Autodesk Inventor part; units mm, degrees
(part 2 of 4)
  line L790 (-24.261051, 21.500592) -> (-24.576272, 21.93055)
  line L791 (-24.576272, 21.93055) -> (-24.635193, 21.981033)
  line L792 (-24.635193, 21.981033) -> (-24.227981, 22.446234)
  line L793 (-24.227981, 22.446234) -> (-22.535064, 20.962239)
  line L794 (-22.535064, 20.962239) -> (-22.945382, 20.499895)
  line L795 (-22.945382, 20.499895) -> (-23.011524, 20.555712)
  line L796 (-23.011524, 20.555712) -> (-23.5045, 20.83708)
  line L797 (-23.5045, 20.83708) -> (-23.53757, 20.838033)
  line L798 (-23.53757, 20.838033) -> (-23.570641, 20.839176)
  line L799 (-23.570641, 20.839176) -> (-23.969586, 20.579524)
  line L800 (-23.969586, 20.579524) -> (-24.016106, 20.525803)
  line L801 (-24.016106, 20.525803) -> (-24.095678, 20.433792)
  line L802 (-24.095678, 20.433792) -> (-22.899891, 19.386042)
  line L803 (-22.899891, 19.386042) -> (-22.46477, 19.882866)
  line L804 (-22.46477, 19.882866) -> (-22.375901, 19.985355)
  line L805 (-22.375901, 19.985355) -> (-22.068949, 20.441221)
  line L806 (-22.068949, 20.441221) -> (-21.949048, 20.82565)
  line L807 (-21.949048, 20.82565) -> (-21.952134, 20.891754)
  line L808 (-21.952134, 20.891754) -> (-21.956287, 20.959)
  line L809 (-21.956287, 20.959) -> (-22.111316, 21.344382)
  line L810 (-22.111316, 21.344382) -> (-22.449282, 21.799296)
  line L811 (-22.449282, 21.799296) -> (-22.543313, 21.900261)
  line L812 (-22.543313, 21.900261) -> (-22.117507, 22.386036)
  line L813 (-22.117507, 22.386036) -> (-20.586859, 21.043582)
  line L814 (-20.586859, 21.043582) -> (-23.801127, 17.377791)
  line L815 (-19.514058, 26.962608) -> (-19.53888, 27.003184)
  line L816 (-19.53888, 27.003184) -> (-19.754869, 27.21483)
  line L817 (-19.754869, 27.21483) -> (-19.772452, 27.217878)
  line L818 (-19.772452, 27.217878) -> (-19.791045, 27.221116)
  line L819 (-19.791045, 27.221116) -> (-20.087673, 27.107388)
  line L820 (-20.087673, 27.107388) -> (-20.127963, 27.08148)
  line L821 (-20.127963, 27.08148) -> (-20.346029, 26.942986)
  line L822 (-20.346029, 26.942986) -> (-20.691234, 27.489722)
  line L823 (-20.691234, 27.489722) -> (-18.695479, 28.747593)
  line L824 (-18.695479, 28.747593) -> (-15.261145, 26.846974)
  line L825 (-15.261145, 26.846974) -> (-16.523017, 28.848939)
  line L826 (-16.523017, 28.848939) -> (-16.547782, 28.889325)
  line L827 (-16.547782, 28.889325) -> (-16.763809, 29.10097)
  line L828 (-16.763809, 29.10097) -> (-16.781336, 29.104209)
  line L829 (-16.781336, 29.104209) -> (-16.800004, 29.107257)
  line L830 (-16.800004, 29.107257) -> (-17.096613, 28.993528)
  line L831 (-17.096613, 28.993528) -> (-17.136999, 28.967621)
  line L832 (-17.136999, 28.967621) -> (-17.3736, 28.817887)
  line L833 (-17.3736, 28.817887) -> (-17.717833, 29.364432)
  line L834 (-17.717833, 29.364432) -> (-15.813024, 30.565534)
  line L835 (-15.813024, 30.565534) -> (-15.46879, 30.018799)
  line L836 (-15.46879, 30.018799) -> (-15.663101, 29.895736)
  line L837 (-15.663101, 29.895736) -> (-15.704439, 29.870209)
  line L838 (-15.704439, 29.870209) -> (-15.934944, 29.652849)
  line L839 (-15.934944, 29.652849) -> (-15.940087, 29.63437)
  line L840 (-15.940087, 29.63437) -> (-15.945231, 29.616844)
  line L841 (-15.945231, 29.616844) -> (-15.84598, 29.331475)
  line L842 (-15.84598, 29.331475) -> (-15.821215, 29.29128)
  line L843 (-15.821215, 29.29128) -> (-13.762482, 26.0263)
  line L844 (-13.762482, 26.0263) -> (-15.043976, 25.218962)
  line L845 (-15.043976, 25.218962) -> (-18.71091, 27.243786)
  line L846 (-18.71091, 27.243786) -> (-17.326165, 25.048654)
  line L847 (-17.326165, 25.048654) -> (-17.30121, 25.009221)
  line L848 (-17.30121, 25.009221) -> (-17.087278, 24.796432)
  line L849 (-17.087278, 24.796432) -> (-17.0688, 24.793385)
  line L850 (-17.0688, 24.793385) -> (-17.051083, 24.790146)
  line L851 (-17.051083, 24.790146) -> (-16.754475, 24.905018)
  line L852 (-16.754475, 24.905018) -> (-16.713136, 24.929783)
  line L853 (-16.713136, 24.929783) -> (-16.476535, 25.079515)
  line L854 (-16.476535, 25.079515) -> (-16.131349, 24.532971)
  line L855 (-16.131349, 24.532971) -> (-18.059781, 23.317391)
  line L856 (-18.059781, 23.317391) -> (-18.405157, 23.864126)
  line L857 (-18.405157, 23.864126) -> (-18.185892, 24.001666)
  line L858 (-18.185892, 24.001666) -> (-18.145696, 24.027575)
  line L859 (-18.145696, 24.027575) -> (-17.914239, 24.245697)
  line L860 (-17.914239, 24.245697) -> (-17.908905, 24.263032)
  line L861 (-17.908905, 24.263032) -> (-17.904904, 24.280749)
  line L862 (-17.904904, 24.280749) -> (-18.003012, 24.56707)
  line L863 (-18.003012, 24.56707) -> (-18.027777, 24.606313)
  line L864 (-18.027777, 24.606313) -> (-19.514058, 26.962608)
  line L865 (-10.748772, 31.507176) -> (-10.761154, 31.552705)
  line L866 (-10.761154, 31.552705) -> (-10.903649, 31.819405)
  line L867 (-10.903649, 31.819405) -> (-10.920222, 31.826454)
  line L868 (-10.920222, 31.826454) -> (-10.936796, 31.835788)
  line L869 (-10.936796, 31.835788) -> (-11.253025, 31.814071)
  line L870 (-11.253025, 31.814071) -> (-11.299507, 31.800546)
  line L871 (-11.299507, 31.800546) -> (-11.549634, 31.73368)
  line L872 (-11.549634, 31.73368) -> (-11.717083, 32.357758)
  line L873 (-11.717083, 32.357758) -> (-9.440418, 32.971549)
  line L874 (-9.440418, 32.971549) -> (-6.717982, 30.143958)
  line L875 (-6.717982, 30.143958) -> (-7.334059, 32.428053)
  line L876 (-7.334059, 32.428053) -> (-7.346442, 32.473392)
  line L877 (-7.346442, 32.473392) -> (-7.488936, 32.740092)
  line L878 (-7.488936, 32.740092) -> (-7.50551, 32.748283)
  line L879 (-7.50551, 32.748283) -> (-7.522083, 32.756665)
  line L880 (-7.522083, 32.756665) -> (-7.838313, 32.734948)
  line L881 (-7.838313, 32.734948) -> (-7.884795, 32.721613)
  line L882 (-7.884795, 32.721613) -> (-8.155495, 32.649033)
  line L883 (-8.155495, 32.649033) -> (-8.324088, 33.273492)
  line L884 (-8.324088, 33.273492) -> (-6.150483, 33.85947)
  line L885 (-6.150483, 33.85947) -> (-5.98189, 33.235201)
  line L886 (-5.98189, 33.235201) -> (-6.203061, 33.175384)
  line L887 (-6.203061, 33.175384) -> (-6.250686, 33.162811)
  line L888 (-6.250686, 33.162811) -> (-6.536055, 33.023365)
  line L889 (-6.536055, 33.023365) -> (-6.545199, 33.007744)
  line L890 (-6.545199, 33.007744) -> (-6.555486, 32.992314)
  line L891 (-6.555486, 32.992314) -> (-6.545199, 32.689609)
  line L892 (-6.545199, 32.689609) -> (-6.532816, 32.64408)
  line L893 (-6.532816, 32.64408) -> (-5.527358, 28.91809)
  line L894 (-5.527358, 28.91809) -> (-6.990779, 28.523375)
  line L895 (-6.990779, 28.523375) -> (-9.897046, 31.540132)
  line L896 (-9.897046, 31.540132) -> (-9.221343, 29.032771)
  line L897 (-9.221343, 29.032771) -> (-9.209913, 28.988575)
  line L898 (-9.209913, 28.988575) -> (-9.066276, 28.721876)
  line L899 (-9.066276, 28.721876) -> (-9.049512, 28.713303)
  line L900 (-9.049512, 28.713303) -> (-9.034272, 28.705111)
  line L901 (-9.034272, 28.705111) -> (-8.717661, 28.726828)
  line L902 (-8.717661, 28.726828) -> (-8.670417, 28.739401)
  line L903 (-8.670417, 28.739401) -> (-8.399526, 28.812553)
  line L904 (-8.399526, 28.812553) -> (-8.230933, 28.188475)
  line L905 (-8.230933, 28.188475) -> (-10.432542, 27.595258)
  line L906 (-10.432542, 27.595258) -> (-10.600753, 28.218384)
  line L907 (-10.600753, 28.218384) -> (-10.35177, 28.286583)
  line L908 (-10.35177, 28.286583) -> (-10.305288, 28.300108)
  line L909 (-10.305288, 28.300108) -> (-10.020109, 28.439554)
  line L910 (-10.020109, 28.439554) -> (-10.009632, 28.454033)
  line L911 (-10.009632, 28.454033) -> (-10.000488, 28.469653)
  line L912 (-10.000488, 28.469653) -> (-10.010775, 28.772358)
  line L913 (-10.010775, 28.772358) -> (-10.022205, 28.816744)
  line L914 (-10.022205, 28.816744) -> (-10.748772, 31.507176)
  line L915 (-1.875853, 29.406151) -> (-1.860232, 30.051946)
  line L916 (-1.860232, 30.051946) -> (-1.587436, 30.04585)
  line L917 (-1.587436, 30.04585) -> (-1.539811, 30.044707)
  line L918 (-1.539811, 30.044707) -> (-1.231963, 30.096333)
  line L919 (-1.231963, 30.096333) -> (-1.217676, 30.107763)
  line L920 (-1.217676, 30.107763) -> (-1.20415, 30.120145)
  line L921 (-1.20415, 30.120145) -> (-1.129855, 30.414658)
  line L922 (-1.129855, 30.414658) -> (-1.128712, 30.46114)
  line L923 (-1.128712, 30.46114) -> (-1.060513, 33.246441)
  line L924 (-1.060513, 33.246441) -> (-1.05937, 33.295209)
  line L925 (-1.05937, 33.295209) -> (-1.119188, 33.594865)
  line L926 (-1.119188, 33.594865) -> (-1.13157, 33.606295)
  line L927 (-1.13157, 33.606295) -> (-1.145095, 33.618678)
  line L928 (-1.145095, 33.618678) -> (-1.451038, 33.683829)
  line L929 (-1.451038, 33.683829) -> (-1.498663, 33.684972)
  line L930 (-1.498663, 33.684972) -> (-1.770316, 33.69202)
  line L931 (-1.770316, 33.69202) -> (-1.754886, 34.337815)
  line L932 (-1.754886, 34.337815) -> (3.119247, 34.217991)
  line L933 (3.119247, 34.217991) -> (3.073718, 32.337184)
  line L934 (3.073718, 32.337184) -> (2.42678, 32.353568)
  line L935 (2.42678, 32.353568) -> (2.418588, 32.425957)
  line L936 (2.418588, 32.425957) -> (2.311908, 32.971549)
  line L937 (2.311908, 32.971549) -> (2.299526, 33.007744)
  line L938 (2.299526, 33.007744) -> (2.286191, 33.045082)
  line L939 (2.286191, 33.045082) -> (2.11055, 33.339595)
  line L940 (2.11055, 33.339595) -> (2.088832, 33.360169)
  line L941 (2.088832, 33.360169) -> (2.066163, 33.383029)
  line L942 (2.066163, 33.383029) -> (1.776603, 33.542097)
  line L943 (1.776603, 33.542097) -> (1.741551, 33.551622)
  line L944 (1.741551, 33.551622) -> (1.705166, 33.561909)
  line L945 (1.705166, 33.561909) -> (1.063561, 33.622678)
  line L946 (1.063561, 33.622678) -> (0.97155, 33.624774)
  line L947 (0.97155, 33.624774) -> (0.332804, 33.640395)
  line L948 (0.332804, 33.640395) -> (0.298704, 32.236791)
  line L949 (0.298704, 32.236791) -> (0.420624, 32.233743)
  line L950 (0.420624, 32.233743) -> (0.48787, 32.2326)
  line L951 (0.48787, 32.2326) -> (0.947737, 32.350519)
  line L952 (0.947737, 32.350519) -> (0.97155, 32.375284)
  line L953 (0.97155, 32.375284) -> (0.994219, 32.401192)
  line L954 (0.994219, 32.401192) -> (1.122426, 32.917828)
  line L955 (1.122426, 32.917828) -> (1.124522, 32.995362)
  line L956 (1.124522, 32.995362) -> (1.742504, 32.980884)
  line L957 (1.742504, 32.980884) -> (1.686687, 30.729936)
  line L958 (1.686687, 30.729936) -> (1.069658, 30.748605)
  line L959 (1.069658, 30.748605) -> (1.069658, 30.83433)
  line L960 (1.069658, 30.83433) -> (0.969455, 31.3944)
  line L961 (0.969455, 31.3944) -> (0.949833, 31.420308)
  line L962 (0.949833, 31.420308) -> (0.929259, 31.446978)
  line L963 (0.929259, 31.446978) -> (0.474345, 31.586805)
  line L964 (0.474345, 31.586805) -> (0.404051, 31.587757)
  line L965 (0.404051, 31.587757) -> (0.28213, 31.590805)
  line L966 (0.28213, 31.590805) -> (0.242888, 30.001273)
  line L967 (0.242888, 30.001273) -> (0.903351, 29.9847)
  line L968 (0.903351, 29.9847) -> (1.038796, 29.981461)
  line L969 (1.038796, 29.981461) -> (1.585341, 30.038421)
  line L970 (1.585341, 30.038421) -> (1.958531, 30.192345)
  line L971 (1.958531, 30.192345) -> (2.007108, 30.237874)
  line L972 (2.007108, 30.237874) -> (2.055876, 30.283404)
  line L973 (2.055876, 30.283404) -> (2.252091, 30.649354)
  line L974 (2.252091, 30.649354) -> (2.384489, 31.20028)
  line L975 (2.384489, 31.20028) -> (2.401824, 31.33744)
  line L976 (2.401824, 31.33744) -> (3.048, 31.3222)
  line L977 (3.048, 31.3222) -> (2.99828, 29.286898)
  line L978 (2.99828, 29.286898) -> (-1.875853, 29.406151)
  line L979 (7.072313, 28.470416) -> (6.501956, 28.644342)
  line L980 (6.501956, 28.644342) -> (7.068312, 30.498478)
  line L981 (7.068312, 30.498478) -> (7.69982, 30.306264)
  line L982 (7.69982, 30.306264) -> (7.685341, 30.207966)
  line L983 (7.685341, 30.207966) -> (7.857935, 29.330332)
  line L984 (7.857935, 29.330332) -> (7.907655, 29.25318)
  line L985 (7.907655, 29.25318) -> (7.956042, 29.176408)
  line L986 (7.956042, 29.176408) -> (8.273605, 28.86437)
  line L987 (8.273605, 28.86437) -> (8.685657, 28.646437)
  line L988 (8.685657, 28.646437) -> (8.782812, 28.616338)
  line L989 (8.782812, 28.616338) -> (8.848916, 28.596717)
  line L990 (8.848916, 28.596717) -> (9.409366, 28.56357)
  line L991 (9.409366, 28.56357) -> (9.454706, 28.577095)
  line L992 (9.454706, 28.577095) -> (9.500045, 28.590621)
  line L993 (9.500045, 28.590621) -> (9.793795, 28.875799)
  line L994 (9.793795, 28.875799) -> (9.807131, 28.919233)
  line L995 (9.807131, 28.919233) -> (9.827895, 28.987432)
  line L996 (9.827895, 28.987432) -> (9.70388, 29.339857)
  line L997 (9.70388, 29.339857) -> (9.27716, 29.705617)
  line L998 (9.27716, 29.705617) -> (9.146667, 29.781246)
  line L999 (9.146667, 29.781246) -> (9.12495, 29.793438)
  line L1000 (9.12495, 29.793438) -> (8.962835, 29.887545)
  line L1001 (8.962835, 29.887545) -> (8.951405, 29.893641)
  line L1002 (8.951405, 29.893641) -> (8.836533, 29.960887)
  line L1003 (8.836533, 29.960887) -> (8.37457, 30.244161)
  line L1004 (8.37457, 30.244161) -> (8.059483, 30.46114)
  line L1005 (8.059483, 30.46114) -> (8.018145, 30.494287)
  line L1006 (8.018145, 30.494287) -> (7.976616, 30.528387)
  line L1007 (7.976616, 30.528387) -> (7.652195, 30.864238)
  line L1008 (7.652195, 30.864238) -> (7.629525, 30.897195)
  line L1009 (7.629525, 30.897195) -> (7.598473, 30.940629)
  line L1010 (7.598473, 30.940629) -> (7.412545, 31.401829)
  line L1011 (7.412545, 31.401829) -> (7.405116, 31.450216)
  line L1012 (7.405116, 31.450216) -> (7.398068, 31.499937)
  line L1013 (7.398068, 31.499937) -> (7.440359, 32.005333)
  line L1014 (7.440359, 32.005333) -> (7.456932, 32.056959)
  line L1015 (7.456932, 32.056959) -> (7.492937, 32.176783)
  line L1016 (7.492937, 32.176783) -> (7.776401, 32.654367)
  line L1017 (7.776401, 32.654367) -> (8.193786, 32.973645)
  line L1018 (8.193786, 32.973645) -> (8.29818, 33.012888)
  line L1019 (8.29818, 33.012888) -> (8.401621, 33.053274)
  line L1020 (8.401621, 33.053274) -> (8.994839, 33.124521)
  line L1021 (8.994839, 33.124521) -> (9.686163, 33.022413)
  line L1022 (9.686163, 33.022413) -> (9.839325, 32.97574)
  line L1023 (9.839325, 32.97574) -> (9.914763, 32.953071)
  line L1024 (9.914763, 32.953071) -> (10.564749, 32.664654)
  line L1025 (10.564749, 32.664654) -> (10.61847, 32.630554)
  line L1026 (10.61847, 32.630554) -> (10.671238, 32.596455)
  line L1027 (10.671238, 32.596455) -> (11.104245, 32.1945)
  line L1028 (11.104245, 32.1945) -> (11.137392, 32.148018)
  line L1029 (11.137392, 32.148018) -> (11.379136, 32.43853)
  line L1030 (11.379136, 32.43853) -> (11.963209, 32.259651)
  line L1031 (11.963209, 32.259651) -> (11.437239, 30.535626)
  line L1032 (11.437239, 30.535626) -> (10.792015, 30.732984)
  line L1033 (10.792015, 30.732984) -> (10.807636, 30.8229)
  line L1034 (10.807636, 30.8229) -> (10.655617, 31.61557)
  line L1035 (10.655617, 31.61557) -> (10.609326, 31.683769)
  line L1036 (10.609326, 31.683769) -> (10.561701, 31.752159)
  line L1037 (10.561701, 31.752159) -> (10.250424, 32.036194)
  line L1038 (10.250424, 32.036194) -> (9.836086, 32.24403)
  line L1039 (9.836086, 32.24403) -> (9.737979, 32.273938)
  line L1040 (9.737979, 32.273938) -> (9.678924, 32.292607)
  line L1041 (9.678924, 32.292607) -> (9.174671, 32.312229)
  line L1042 (9.174671, 32.312229) -> (9.133332, 32.297751)
  line L1043 (9.133332, 32.297751) -> (9.09085, 32.284416)
  line L1044 (9.09085, 32.284416) -> (8.818054, 32.00419)
  line L1045 (8.818054, 32.00419) -> (8.805672, 31.9619)
  line L1046 (8.805672, 31.9619) -> (8.787003, 31.901892)
  line L1047 (8.787003, 31.901892) -> (8.939974, 31.571184)
  line L1048 (8.939974, 31.571184) -> (9.420416, 31.202376)
  line L1049 (9.420416, 31.202376) -> (9.566339, 31.121604)
  line L1050 (9.566339, 31.121604) -> (9.621012, 31.091695)
  line L1051 (9.621012, 31.091695) -> (10.056304, 30.843474)
  line L1052 (10.056304, 30.843474) -> (10.088309, 30.824043)
  line L1053 (10.088309, 30.824043) -> (10.212324, 30.749557)
  line L1054 (10.212324, 30.749557) -> (11.055667, 29.97327)
  line L1055 (11.055667, 29.97327) -> (11.100054, 29.891736)
  line L1056 (11.100054, 29.891736) -> (11.143488, 29.811155)
  line L1057 (11.143488, 29.811155) -> (11.25093, 29.377957)
  line L1058 (11.25093, 29.377957) -> (11.210734, 28.908947)
  line L1059 (11.210734, 28.908947) -> (11.180826, 28.808553)
  line L1060 (11.180826, 28.808553) -> (11.144441, 28.691586)
  line L1061 (11.144441, 28.691586) -> (10.856214, 28.217241)
  line L1062 (10.856214, 28.217241) -> (10.42016, 27.891867)
  line L1063 (10.42016, 27.891867) -> (10.311575, 27.849576)
  line L1064 (10.311575, 27.849576) -> (10.202037, 27.807095)
  line L1065 (10.202037, 27.807095) -> (9.596437, 27.727465)
  line L1066 (9.596437, 27.727465) -> (8.90797, 27.824621)
  line L1067 (8.90797, 27.824621) -> (8.758238, 27.87015)
  line L1068 (8.758238, 27.87015) -> (8.685657, 27.89282)
  line L1069 (8.685657, 27.89282) -> (8.013954, 28.202001)
  line L1070 (8.013954, 28.202001) -> (7.952041, 28.241053)
  line L1071 (7.952041, 28.241053) -> (7.888795, 28.28163)
  line L1072 (7.888795, 28.28163) -> (7.401115, 28.710446)
  line L1073 (7.401115, 28.710446) -> (7.366064, 28.755975)
  line L1074 (7.366064, 28.755975) -> (7.072313, 28.470416)
  line L1075 (14.207871, 25.663588) -> (13.702474, 25.979628)
  line L1076 (13.702474, 25.979628) -> (14.731937, 27.623071)
  line L1077 (14.731937, 27.623071) -> (15.292197, 27.271599)
  line L1078 (15.292197, 27.271599) -> (15.252001, 27.18073)
  line L1079 (15.252001, 27.18073) -> (15.190851, 26.288809)
  line L1080 (15.190851, 26.288809) -> (15.218855, 26.201942)
  line L1081 (15.218855, 26.201942) -> (15.245524, 26.115264)
  line L1082 (15.245524, 26.115264) -> (15.471076, 25.730644)
  line L1083 (15.471076, 25.730644) -> (15.812072, 25.412509)
  line L1084 (15.812072, 25.412509) -> (15.897797, 25.358788)
  line L1085 (15.897797, 25.358788) -> (15.956852, 25.322403)
  line L1086 (15.956852, 25.322403) -> (16.487775, 25.144666)
  line L1087 (16.487775, 25.144666) -> (16.5354, 25.145809)
  line L1088 (16.5354, 25.145809) -> (16.583025, 25.147905)
  line L1089 (16.583025, 25.147905) -> (16.940403, 25.346215)
  line L1090 (16.940403, 25.346215) -> (16.965359, 25.384315)
  line L1091 (16.965359, 25.384315) -> (17.002697, 25.445466)
  line L1092 (17.002697, 25.445466) -> (16.974693, 25.817513)
  line L1093 (16.974693, 25.817513) -> (16.658463, 26.282713)
  line L1094 (16.658463, 26.282713) -> (16.552164, 26.389013)
  line L1095 (16.552164, 26.389013) -> (16.534257, 26.406729)
  line L1096 (16.534257, 26.406729) -> (16.400907, 26.540079)
  line L1097 (16.400907, 26.540079) -> (16.392716, 26.54827)
  line L1098 (16.392716, 26.54827) -> (16.299561, 26.642187)
  line L1099 (16.299561, 26.642187) -> (15.927705, 27.037284)
  line L1100 (15.927705, 27.037284) -> (15.678722, 27.328558)
  line L1101 (15.678722, 27.328558) -> (15.64767, 27.37085)
  line L1102 (15.64767, 27.37085) -> (15.615666, 27.414283)
  line L1103 (15.615666, 27.414283) -> (15.390305, 27.823668)
  line L1104 (15.390305, 27.823668) -> (15.376779, 27.863101)
  line L1105 (15.376779, 27.863101) -> (15.359253, 27.912441)
  line L1106 (15.359253, 27.912441) -> (15.299245, 28.405455)
  line L1107 (15.299245, 28.405455) -> (15.305532, 28.454033)
  line L1108 (15.305532, 28.454033) -> (15.310675, 28.503562)
  line L1109 (15.310675, 28.503562) -> (15.484221, 28.981146)
  line L1110 (15.484221, 28.981146) -> (15.513367, 29.026676)
  line L1111 (15.513367, 29.026676) -> (15.579471, 29.132022)
  line L1112 (15.579471, 29.132022) -> (15.976283, 29.519499)
  line L1113 (15.976283, 29.519499) -> (16.463201, 29.719143)
  line L1114 (16.463201, 29.719143) -> (16.574834, 29.730382)
  line L1115 (16.574834, 29.730382) -> (16.685514, 29.742955)
  line L1116 (16.685514, 29.742955) -> (17.276445, 29.65723)
  line L1117 (17.276445, 29.65723) -> (17.916335, 29.377005)
  line L1118 (17.916335, 29.377005) -> (18.05178, 29.292232)
  line L1119 (18.05178, 29.292232) -> (18.118646, 29.249941)
  line L1120 (18.118646, 29.249941) -> (18.670524, 28.804362)
  line L1121 (18.670524, 28.804362) -> (18.713958, 28.757118)
  line L1122 (18.713958, 28.757118) -> (18.75663, 28.710446)
  line L1123 (18.75663, 28.710446) -> (19.070574, 28.208097)
  line L1124 (19.070574, 28.208097) -> (19.090196, 28.154376)
  line L1125 (19.090196, 28.154376) -> (19.399187, 28.372308)
  line L1126 (19.399187, 28.372308) -> (19.916966, 28.047886)
  line L1127 (19.916966, 28.047886) -> (18.960084, 26.520267)
  line L1128 (18.960084, 26.520267) -> (18.387441, 26.878978)
  line L1129 (18.387441, 26.878978) -> (18.426875, 26.961655)
  line L1130 (18.426875, 26.961655) -> (18.486692, 27.766708)
  line L1131 (18.486692, 27.766708) -> (18.460022, 27.844242)
  line L1132 (18.460022, 27.844242) -> (18.432018, 27.922728)
  line L1133 (18.432018, 27.922728) -> (17.859375, 28.587382)
  line L1134 (17.859375, 28.587382) -> (17.772507, 28.642247)
  line L1135 (17.772507, 28.642247) -> (17.719929, 28.675203)
  line L1136 (17.719929, 28.675203) -> (17.237012, 28.825126)
  line L1137 (17.237012, 28.825126) -> (17.193768, 28.822078)
  line L1138 (17.193768, 28.822078) -> (17.149191, 28.819983)
  line L1139 (17.149191, 28.819983) -> (16.81353, 28.619386)
  line L1140 (16.81353, 28.619386) -> (16.79067, 28.582049)
  line L1141 (16.79067, 28.582049) -> (16.75657, 28.52947)
  line L1142 (16.75657, 28.52947) -> (16.818483, 28.170949)
  line L1143 (16.818483, 28.170949) -> (17.186529, 27.689175)
  line L1144 (17.186529, 27.689175) -> (17.306354, 27.573541)
  line L1145 (17.306354, 27.573541) -> (17.350931, 27.530107)
  line L1146 (17.350931, 27.530107) -> (17.705451, 27.17673)
  line L1147 (17.705451, 27.17673) -> (17.731359, 27.149679)
  line L1148 (17.731359, 27.149679) -> (17.832324, 27.045475)
  line L1149 (17.832324, 27.045475) -> (18.218849, 26.546175)
  line L1150 (18.218849, 26.546175) -> (18.445353, 26.077164)
  line L1151 (18.445353, 26.077164) -> (18.46707, 25.987057)
  line L1152 (18.46707, 25.987057) -> (18.487835, 25.898284)
  line L1153 (18.487835, 25.898284) -> (18.317147, 25.008459)
  line L1154 (18.317147, 25.008459) -> (18.262283, 24.919495)
  line L1155 (18.262283, 24.919495) -> (18.197322, 24.816054)
  line L1156 (18.197322, 24.816054) -> (17.794224, 24.43372)
  line L1157 (17.794224, 24.43372) -> (17.289971, 24.234267)
  line L1158 (17.289971, 24.234267) -> (17.174147, 24.220741)
  line L1159 (17.174147, 24.220741) -> (17.05737, 24.208359)
  line L1160 (17.05737, 24.208359) -> (16.450818, 24.288941)
  line L1161 (16.450818, 24.288941) -> (15.810929, 24.561737)
  line L1162 (15.810929, 24.561737) -> (15.678722, 24.644604)
  line L1163 (15.678722, 24.644604) -> (15.614713, 24.684799)
  line L1164 (15.614713, 24.684799) -> (15.047214, 25.158192)
  line L1165 (15.047214, 25.158192) -> (14.997684, 25.212865)
  line L1166 (14.997684, 25.212865) -> (14.94682, 25.267729)
  line L1167 (14.94682, 25.267729) -> (14.587347, 25.810273)
  line L1168 (14.587347, 25.810273) -> (14.56563, 25.863042)
  line L1169 (14.56563, 25.863042) -> (14.207871, 25.663588)
  line L1170 (19.891439, 21.741384) -> (20.367688, 22.178391)
  line L1171 (20.367688, 22.178391) -> (20.551712, 21.977032)
  line L1172 (20.551712, 21.977032) -> (20.583716, 21.94198)
  line L1173 (20.583716, 21.94198) -> (20.834795, 21.756624)
  line L1174 (20.834795, 21.756624) -> (20.853464, 21.754909)
  line L1175 (20.853464, 21.754909) -> (20.87118, 21.752623)
  line L1176 (20.87118, 21.752623) -> (21.135785, 21.902547)
  line L1177 (21.135785, 21.902547) -> (21.170836, 21.934551)
  line L1178 (21.170836, 21.934551) -> (23.224236, 23.815738)
  line L1179 (23.224236, 23.815738) -> (23.259479, 23.848695)
  line L1180 (23.259479, 23.848695) -> (23.433024, 24.098821)
  line L1181 (23.433024, 24.098821) -> (23.433024, 24.116157)
  line L1182 (23.433024, 24.116157) -> (23.432262, 24.135016)
  line L1183 (23.432262, 24.135016) -> (23.268813, 24.400764)
  line L1184 (23.268813, 24.400764) -> (23.236809, 24.435626)
  line L1185 (23.236809, 24.435626) -> (23.052786, 24.636222)
  line L1186 (23.052786, 24.636222) -> (23.529417, 25.072467)
  line L1187 (23.529417, 25.072467) -> (26.82221, 21.476779)
  line L1188 (26.82221, 21.476779) -> (25.434036, 20.206525)
  line L1189 (25.434036, 20.206525) -> (24.997791, 20.682966)
  line L1190 (24.997791, 20.682966) -> (25.043321, 20.739925)
  line L1191 (25.043321, 20.739925) -> (25.362598, 21.194458)
  line L1192 (25.362598, 21.194458) -> (25.381458, 21.229701)
  line L1193 (25.381458, 21.229701) -> (25.398984, 21.264753)
  line L1194 (25.398984, 21.264753) -> (25.4889, 21.594508)
  line L1195 (25.4889, 21.594508) -> (25.490043, 21.624417)
  line L1196 (25.490043, 21.624417) -> (25.490043, 21.656611)
  line L1197 (25.490043, 21.656611) -> (25.404318, 21.97608)
  line L1198 (25.404318, 21.97608) -> (25.386602, 22.008084)
  line L1199 (25.386602, 22.008084) -> (25.369076, 22.04104)
  line L1200 (25.369076, 22.04104) -> (24.96693, 22.545484)
  line L1201 (24.96693, 22.545484) -> (24.905018, 22.613683)
  line L1202 (24.905018, 22.613683) -> (24.473916, 23.08498)
  line L1203 (24.473916, 23.08498) -> (23.438358, 22.137243)
  line L1204 (23.438358, 22.137243) -> (23.520083, 22.047136)
  line L1205 (23.520083, 22.047136) -> (23.565422, 21.997797)
  line L1206 (23.565422, 21.997797) -> (23.96852, 21.74748)
  line L1207 (23.96852, 21.74748) -> (24.003762, 21.74748)
  line L1208 (24.003762, 21.74748) -> (24.037862, 21.748432)
  line L1209 (24.037862, 21.748432) -> (24.500967, 22.015132)
  line L1210 (24.500967, 22.015132) -> (24.558688, 22.067901)
  line L1211 (24.558688, 22.067901) -> (24.975312, 21.612225)
  line L1212 (24.975312, 21.612225) -> (23.314343, 20.091844)
  line L1213 (23.314343, 20.091844) -> (22.900958, 20.549616)
  line L1214 (22.900958, 20.549616) -> (22.96287, 20.608671)
  line L1215 (22.96287, 20.608671) -> (23.295673, 21.068538)
  line L1216 (23.295673, 21.068538) -> (23.300817, 21.101494)
  line L1217 (23.300817, 21.101494) -> (23.305008, 21.134641)
  line L1218 (23.305008, 21.134641) -> (23.092029, 21.558313)
  line L1219 (23.092029, 21.558313) -> (23.044595, 21.610129)
  line L1220 (23.044595, 21.610129) -> (22.960775, 21.700045)
  line L1221 (22.960775, 21.700045) -> (21.789009, 20.626197)
  line L1222 (21.789009, 20.626197) -> (22.234208, 20.139279)
  line L1223 (22.234208, 20.139279) -> (22.325267, 20.040028)
  line L1224 (22.325267, 20.040028) -> (22.744938, 19.685508)
  line L1225 (22.744938, 19.685508) -> (23.114889, 19.523392)
  line L1226 (23.114889, 19.523392) -> (23.181945, 19.519011)
  line L1227 (23.181945, 19.519011) -> (23.248239, 19.516153)
  line L1228 (23.248239, 19.516153) -> (23.647146, 19.628929)
  line L1229 (23.647146, 19.628929) -> (24.137112, 19.915251)
  line L1230 (24.137112, 19.915251) -> (24.248555, 19.997737)
  line L1231 (24.248555, 19.997737) -> (24.685943, 19.520154)
  line L1232 (24.685943, 19.520154) -> (23.18404, 18.145696)
  line L1233 (23.18404, 18.145696) -> (19.891439, 21.741384)
  line L1234 (25.152096, 15.362491) -> (25.731788, 15.649575)
  line L1235 (25.731788, 15.649575) -> (25.852755, 15.404782)
  line L1236 (25.852755, 15.404782) -> (25.873329, 15.362491)
  line L1237 (25.873329, 15.362491) -> (26.062495, 15.11427)
  line L1238 (26.062495, 15.11427) -> (26.080022, 15.107221)
  line L1239 (26.080022, 15.107221) -> (26.096595, 15.100744)
  line L1240 (26.096595, 15.100744) -> (26.392251, 15.172182)
  line L1241 (26.392251, 15.172182) -> (26.434542, 15.192946)
  line L1242 (26.434542, 15.192946) -> (28.930663, 16.430053)
  line L1243 (28.930663, 16.430053) -> (28.972954, 16.45177)
  line L1244 (28.972954, 16.45177) -> (29.209556, 16.644937)
  line L1245 (29.209556, 16.644937) -> (29.214699, 16.661701)
  line L1246 (29.214699, 16.661701) -> (29.219081, 16.679037)
  line L1247 (29.219081, 16.679037) -> (29.134117, 16.979836)
  line L1248 (29.134117, 16.979836) -> (29.113353, 17.022318)
  line L1249 (29.113353, 17.022318) -> (28.992576, 17.267301)
  line L1250 (28.992576, 17.267301) -> (29.571505, 17.554575)
  line L1251 (29.571505, 17.554575) -> (31.73749, 13.185838)
  line L1252 (31.73749, 13.185838) -> (30.052899, 12.350686)
  line L1253 (30.052899, 12.350686) -> (29.765625, 12.929425)
  line L1254 (29.765625, 12.929425) -> (29.82468, 12.970573)
  line L1255 (29.82468, 12.970573) -> (30.258639, 13.319188)
  line L1256 (30.258639, 13.319188) -> (30.2855, 13.347001)
  line L1257 (30.2855, 13.347001) -> (30.312169, 13.375957)
  line L1258 (30.312169, 13.375957) -> (30.488954, 13.668375)
  line L1259 (30.488954, 13.668375) -> (30.498479, 13.697521)
  line L1260 (30.498479, 13.697521) -> (30.507813, 13.72743)
  line L1261 (30.507813, 13.72743) -> (30.513909, 14.058138)
  line L1262 (30.513909, 14.058138) -> (30.50667, 14.094333)
  line L1263 (30.50667, 14.094333) -> (30.498479, 14.130337)
  line L1264 (30.498479, 14.130337) -> (30.252543, 14.726793)
  line L1265 (30.252543, 14.726793) -> (30.211204, 14.80947)
  line L1266 (30.211204, 14.80947) -> (29.92774, 15.382113)
  line L1267 (29.92774, 15.382113) -> (28.67006, 14.758797)
  line L1268 (28.67006, 14.758797) -> (28.723971, 14.649259)
  line L1269 (28.723971, 14.649259) -> (28.753879, 14.588299)
  line L1270 (28.753879, 14.588299) -> (29.072205, 14.235874)
  line L1271 (29.072205, 14.235874) -> (29.106305, 14.22673)
  line L1272 (29.106305, 14.22673) -> (29.139261, 14.218158)
  line L1273 (29.139261, 14.218158) -> (29.656087, 14.346555)
  line L1274 (29.656087, 14.346555) -> (29.726382, 14.380654)
  line L1275 (29.726382, 14.380654) -> (30.001274, 13.827633)
  line L1276 (30.001274, 13.827633) -> (27.983878, 12.826936)
  line L1277 (27.983878, 12.826936) -> (27.712988, 13.382053)
  line L1278 (27.712988, 13.382053) -> (27.788425, 13.422249)
  line L1279 (27.788425, 13.422249) -> (28.236101, 13.770673)
  line L1280 (28.236101, 13.770673) -> (28.250388, 13.800582)
  line L1281 (28.250388, 13.800582) -> (28.263913, 13.831633)
  line L1282 (28.263913, 13.831633) -> (28.176093, 14.29893)
  line L1283 (28.176093, 14.29893) -> (28.145041, 14.361795)
  line L1284 (28.145041, 14.361795) -> (28.090368, 14.471332)
  line L1285 (28.090368, 14.471332) -> (26.666, 13.764387)
  line L1286 (26.666, 13.764387) -> (26.95975, 13.173265)
  line L1287 (26.95975, 13.173265) -> (27.019567, 13.052488)
  line L1288 (27.019567, 13.052488) -> (27.323606, 12.595479)
  line L1289 (27.323606, 12.595479) -> (27.634501, 12.337161)
  line L1290 (27.634501, 12.337161) -> (27.697557, 12.314491)
  line L1291 (27.697557, 12.314491) -> (27.760612, 12.292774)
  line L1292 (27.760612, 12.292774) -> (28.176093, 12.289726)
  line L1293 (28.176093, 12.289726) -> (28.724733, 12.429363)
  line L1294 (28.724733, 12.429363) -> (28.855225, 12.47775)
  line L1295 (28.855225, 12.47775) -> (29.1425, 11.899201)
  line L1296 (29.1425, 11.899201) -> (27.319224, 10.994707)
  line L1297 (27.319224, 10.994707) -> (25.152096, 15.362491)
  line L1298 (-9.504426, -27.822582) -> (-10.266045, -29.566152)
  line L1299 (-10.266045, -29.566152) -> (-10.876788, -29.29951)
  line L1300 (-10.876788, -29.29951) -> (-10.834497, -29.202355)
  line L1301 (-10.834497, -29.202355) -> (-10.711434, -28.768281)
  line L1302 (-10.711434, -28.768281) -> (-10.704195, -28.404483)
  line L1303 (-10.704195, -28.404483) -> (-10.719816, -28.342457)
  line L1304 (-10.719816, -28.342457) -> (-10.736199, -28.279401)
  line L1305 (-10.736199, -28.279401) -> (-10.90803, -28.01173)
  line L1306 (-10.90803, -28.01173) -> (-11.199305, -27.802942)
  line L1307 (-11.199305, -27.802942) -> (-11.274742, -27.769871)
  line L1308 (-11.274742, -27.769871) -> (-11.344084, -27.739905)
  line L1309 (-11.344084, -27.739905) -> (-12.598718, -30.612074)
  line L1310 (-12.598718, -30.612074) -> (-12.616243, -30.650307)
  line L1311 (-12.616243, -30.650307) -> (-12.708255, -30.915959)
  line L1312 (-12.708255, -30.915959) -> (-12.709398, -30.930399)
  line L1313 (-12.709398, -30.930399) -> (-12.711303, -30.943848)
  line L1314 (-12.711303, -30.943848) -> (-12.674155, -31.053405)
  line L1315 (-12.674155, -31.053405) -> (-12.664821, -31.061654)
  line L1316 (-12.664821, -31.061654) -> (-12.655486, -31.070969)
  line L1317 (-12.655486, -31.070969) -> (-12.51604, -31.174315)
  line L1318 (-12.51604, -31.174315) -> (-12.496419, -31.185688)
  line L1319 (-12.496419, -31.185688) -> (-12.47775, -31.196013)
  line L1320 (-12.47775, -31.196013) -> (-12.136755, -31.364511)
  line L1321 (-12.136755, -31.364511) -> (-12.087034, -31.388266)
  line L1322 (-12.087034, -31.388266) -> (-12.339256, -31.967043)
  line L1323 (-12.339256, -31.967043) -> (-15.021306, -30.797068)
  line L1324 (-15.021306, -30.797068) -> (-14.769084, -30.217262)
  line L1325 (-14.769084, -30.217262) -> (-14.734032, -30.23174)
  line L1326 (-14.734032, -30.23174) -> (-14.425994, -30.351622)
  line L1327 (-14.425994, -30.351622) -> (-14.399133, -30.360937)
  line L1328 (-14.399133, -30.360937) -> (-14.373225, -30.369186)
  line L1329 (-14.373225, -30.369186) -> (-14.145958, -30.420888)
  line L1330 (-14.145958, -30.420888) -> (-14.126337, -30.422964)
  line L1331 (-14.126337, -30.422964) -> (-14.114907, -30.423993)
  line L1332 (-14.114907, -30.423993) -> (-14.012608, -30.376444)
  line L1333 (-14.012608, -30.376444) -> (-14.003274, -30.3661)
  line L1334 (-14.003274, -30.3661) -> (-13.993939, -30.354746)
  line L1335 (-13.993939, -30.354746) -> (-13.865733, -30.111859)
  line L1336 (-13.865733, -30.111859) -> (-13.84935, -30.074654)
  line L1337 (-13.84935, -30.074654) -> (-13.809916, -29.984719)
  line L1338 (-13.809916, -29.984719) -> (-12.591478, -27.195247)
  line L1339 (-12.591478, -27.195247) -> (-12.656629, -27.16631)
  line L1340 (-12.656629, -27.16631) -> (-12.734163, -27.13221)
  line L1341 (-12.734163, -27.13221) -> (-13.405866, -27.117732)
  line L1342 (-13.405866, -27.117732) -> (-13.462825, -27.148746)
  line L1343 (-13.462825, -27.148746) -> (-13.520547, -27.178711)
  line L1344 (-13.520547, -27.178711) -> (-14.017752, -27.812257)
  line L1345 (-14.017752, -27.812257) -> (-14.05909, -27.909412)
  line L1346 (-14.05909, -27.909412) -> (-14.66469, -27.645855)
  line L1347 (-14.66469, -27.645855) -> (-13.903071, -25.901256)
  line L1348 (-13.903071, -25.901256) -> (-9.504426, -27.822582)
  line L1349 (-7.424737, -33.519408) -> (-7.334059, -32.879633)
  line L1350 (-7.334059, -32.879633) -> (-7.064121, -32.917905)
  line L1351 (-7.064121, -32.917905) -> (-7.016686, -32.924096)
  line L1352 (-7.016686, -32.924096) -> (-6.704457, -32.907561)
  line L1353 (-6.704457, -32.907561) -> (-6.688836, -32.898245)
  line L1354 (-6.688836, -32.898245) -> (-6.674549, -32.88792)
  line L1355 (-6.674549, -32.88792) -> (-6.565963, -32.604742)
  line L1356 (-6.565963, -32.604742) -> (-6.558725, -32.558222)
  line L1357 (-6.558725, -32.558222) -> (-6.168961, -29.799724)
  line L1358 (-6.168961, -29.799724) -> (-6.162865, -29.752176)
  line L1359 (-6.162865, -29.752176) -> (-6.187821, -29.447299)
  line L1360 (-6.187821, -29.447299) -> (-6.199251, -29.433869)
  line L1361 (-6.199251, -29.433869) -> (-6.211633, -29.42042)
  line L1362 (-6.211633, -29.42042) -> (-6.506146, -29.319131)
  line L1363 (-6.506146, -29.319131) -> (-6.553771, -29.312959)
  line L1364 (-6.553771, -29.312959) -> (-6.823329, -29.274687)
  line L1365 (-6.823329, -29.274687) -> (-6.73227, -28.63495)
  line L1366 (-6.73227, -28.63495) -> (-1.904809, -29.318102)
  line L1367 (-1.904809, -29.318102) -> (-2.169414, -31.181573)
  line L1368 (-2.169414, -31.181573) -> (-2.809113, -31.09061)
  line L1369 (-2.809113, -31.09061) -> (-2.809113, -30.924208)
  line L1370 (-2.809113, -30.924208) -> (-2.850261, -30.463255)
  line L1371 (-2.850261, -30.463255) -> (-2.858833, -30.425022)
  line L1372 (-2.858833, -30.425022) -> (-2.868168, -30.386788)
  line L1373 (-2.868168, -30.386788) -> (-3.008566, -30.075683)
  line L1374 (-3.008566, -30.075683) -> (-3.027045, -30.051908)
  line L1375 (-3.027045, -30.051908) -> (-3.046857, -30.027105)
  line L1376 (-3.046857, -30.027105) -> (-3.316605, -29.834872)
  line L1377 (-3.316605, -29.834872) -> (-3.350704, -29.821422)
  line L1378 (-3.350704, -29.821422) -> (-3.384804, -29.806944)
  line L1379 (-3.384804, -29.806944) -> (-4.016311, -29.671575)
  line L1380 (-4.016311, -29.671575) -> (-4.10718, -29.659174)
  line L1381 (-4.10718, -29.659174) -> (-4.73983, -29.570286)
  line L1382 (-4.73983, -29.570286) -> (-4.937189, -30.960384)
  line L1383 (-4.937189, -30.960384) -> (-4.816221, -30.976919)
  line L1384 (-4.816221, -30.976919) -> (-4.748975, -30.986235)
  line L1385 (-4.748975, -30.986235) -> (-4.27882, -30.923179)
  line L1386 (-4.27882, -30.923179) -> (-4.251769, -30.901481)
  line L1387 (-4.251769, -30.901481) -> (-4.226243, -30.878736)
  line L1388 (-4.226243, -30.878736) -> (-4.039171, -30.37953)
  line L1389 (-4.039171, -30.37953) -> (-4.027741, -30.302016)
  line L1390 (-4.027741, -30.302016) -> (-3.415855, -30.387817)
  line L1391 (-3.415855, -30.387817) -> (-3.731895, -32.617124)
  line L1392 (-3.731895, -32.617124) -> (-4.342828, -32.527208)
  line L1393 (-4.342828, -32.527208) -> (-4.332541, -32.441445)
  line L1394 (-4.332541, -32.441445) -> (-4.367784, -31.87507)
  line L1395 (-4.367784, -31.87507) -> (-4.384167, -31.847161)
  line L1396 (-4.384167, -31.847161) -> (-4.401883, -31.818205)
  line L1397 (-4.401883, -31.818205) -> (-4.837938, -31.62702)
  line L1398 (-4.837938, -31.62702) -> (-4.90728, -31.617704)
  line L1399 (-4.90728, -31.617704) -> (-5.028057, -31.60014)
  line L1400 (-5.028057, -31.60014) -> (-5.25037, -33.175232)
  line L1401 (-5.25037, -33.175232) -> (-4.596003, -33.267225)
  line L1402 (-4.596003, -33.267225) -> (-4.462653, -33.285836)
  line L1403 (-4.462653, -33.285836) -> (-3.914013, -33.292028)
  line L1404 (-3.914013, -33.292028) -> (-3.525393, -33.183519)
  line L1405 (-3.525393, -33.183519) -> (-3.471672, -33.144219)
  line L1406 (-3.471672, -33.144219) -> (-3.417951, -33.103928)
  line L1407 (-3.417951, -33.103928) -> (-3.180207, -32.762857)
  line L1408 (-3.180207, -32.762857) -> (-2.983611, -32.231628)
  line L1409 (-2.983611, -32.231628) -> (-2.950655, -32.097269)
  line L1410 (-2.950655, -32.097269) -> (-2.310955, -32.187166)
  line L1411 (-2.310955, -32.187166) -> (-2.596134, -34.203589)
  line L1412 (-2.596134, -34.203589) -> (-7.424737, -33.519408)
  line L1413 (5.837492, -31.82855) -> (6.61035, -31.72728)
  line L1414 (6.61035, -31.72728) -> (6.626923, -31.895739)
  line L1415 (6.626923, -31.895739) -> (6.568059, -32.634688)
  line L1416 (6.568059, -32.634688) -> (6.313742, -33.231049)
  line L1417 (6.313742, -33.231049) -> (6.234303, -33.329213)
  line L1418 (6.234303, -33.329213) -> (6.153722, -33.426368)
  line L1419 (6.153722, -33.426368) -> (5.610034, -33.802587)
  line L1420 (5.610034, -33.802587) -> (4.875276, -34.029968)
  line L1421 (4.875276, -34.029968) -> (4.700587, -34.053723)
  line L1422 (4.700587, -34.053723) -> (4.502087, -34.079574)
  line L1423 (4.502087, -34.079574) -> (3.60807, -34.017566)
  line L1424 (3.60807, -34.017566) -> (2.845308, -33.700269)
  line L1425 (2.845308, -33.700269) -> (2.711958, -33.59898)
  line L1426 (2.711958, -33.59898) -> (2.578608, -33.496682)
  line L1427 (2.578608, -33.496682) -> (2.072259, -32.844505)
  line L1428 (2.072259, -32.844505) -> (1.781747, -32.000114)
  line L1429 (1.781747, -32.000114) -> (1.756029, -31.802699)
  line L1430 (1.756029, -31.802699) -> (1.742504, -31.703486)
  line L1431 (1.742504, -31.703486) -> (1.777746, -30.802269)
  line L1432 (1.777746, -30.802269) -> (1.79832, -30.720621)
  line L1433 (1.79832, -30.720621) -> (1.817941, -30.638953)
  line L1434 (1.817941, -30.638953) -> (2.190941, -29.877258)
  line L1435 (2.190941, -29.877258) -> (2.245805, -29.806944)
  line L1436 (2.245805, -29.806944) -> (2.298764, -29.739774)
  line L1437 (2.298764, -29.739774) -> (2.906268, -29.215804)
  line L1438 (2.906268, -29.215804) -> (2.97542, -29.178561)
  line L1439 (2.97542, -29.178561) -> (3.043809, -29.140328)
  line L1440 (3.043809, -29.140328) -> (3.861245, -28.891249)
  line L1441 (3.861245, -28.891249) -> (3.956304, -28.879876)
  line L1442 (3.956304, -28.879876) -> (4.022408, -28.870599)
  line L1443 (4.022408, -28.870599) -> (4.659059, -28.884029)
  line L1444 (4.659059, -28.884029) -> (4.720209, -28.896412)
  line L1445 (4.720209, -28.896412) -> (4.780979, -28.907784)
  line L1446 (4.780979, -28.907784) -> (5.382768, -29.13105)
  line L1447 (5.382768, -29.13105) -> (5.442395, -29.164121)
  line L1448 (5.442395, -29.164121) -> (5.537645, -28.756908)
  line L1449 (5.537645, -28.756908) -> (6.206299, -28.66905)
  line L1450 (6.206299, -28.66905) -> (6.469952, -30.662728)
  line L1451 (6.469952, -30.662728) -> (5.753671, -30.757806)
  line L1452 (5.753671, -30.757806) -> (5.731955, -30.651374)
  line L1453 (5.731955, -30.651374) -> (5.564505, -30.19867)
  line L1454 (5.564505, -30.19867) -> (5.315522, -29.854493)
  line L1455 (5.315522, -29.854493) -> (5.253228, -29.801801)
  line L1456 (5.253228, -29.801801) -> (5.190363, -29.74909)
  line L1457 (5.190363, -29.74909) -> (4.837938, -29.581659)
  line L1458 (4.837938, -29.581659) -> (4.431792, -29.543426)
  line L1459 (4.431792, -29.543426) -> (4.342829, -29.555808)
  line L1460 (4.342829, -29.555808) -> (4.244721, -29.56821)
  line L1461 (4.244721, -29.56821) -> (3.835337, -29.747032)
  line L1462 (3.835337, -29.747032) -> (3.533585, -30.077759)
  line L1463 (3.533585, -30.077759) -> (3.490151, -30.166628)
  line L1464 (3.490151, -30.166628) -> (3.445574, -30.255534)
  line L1465 (3.445574, -30.255534) -> (3.320796, -30.787791)
  line L1466 (3.320796, -30.787791) -> (3.322892, -31.437872)
  line L1467 (3.322892, -31.437872) -> (3.342513, -31.585662)
  line L1468 (3.342513, -31.585662) -> (3.362135, -31.735528)
  line L1469 (3.362135, -31.735528) -> (3.528441, -32.372198)
  line L1470 (3.528441, -32.372198) -> (3.785997, -32.854849)
  line L1471 (3.785997, -32.854849) -> (3.850958, -32.929239)
  line L1472 (3.850958, -32.929239) -> (3.914966, -33.002639)
  line L1473 (3.914966, -33.002639) -> (4.293489, -33.241374)
  line L1474 (4.293489, -33.241374) -> (4.741926, -33.305458)
  line L1475 (4.741926, -33.305458) -> (4.843272, -33.292028)
  line L1476 (4.843272, -33.292028) -> (4.927854, -33.280674)
  line L1477 (4.927854, -33.280674) -> (5.291709, -33.145247)
  line L1478 (5.291709, -33.145247) -> (5.572887, -32.901369)
  line L1479 (5.572887, -32.901369) -> (5.617083, -32.837285)
  line L1480 (5.617083, -32.837285) -> (5.660707, -32.772172)
  line L1481 (5.660707, -32.772172) -> (5.803392, -32.390791)
  line L1482 (5.803392, -32.390791) -> (5.843588, -31.931896)
  line L1483 (5.843588, -31.931896) -> (5.837492, -31.82855)
  line L1484 (11.182922, -32.486917) -> (10.920222, -31.895739)
  line L1485 (10.920222, -31.895739) -> (11.170349, -31.785135)
  line L1486 (11.170349, -31.785135) -> (11.213783, -31.765513)
  line L1487 (11.213783, -31.765513) -> (11.470196, -31.586691)
  line L1488 (11.470196, -31.586691) -> (11.478387, -31.571203)
  line L1489 (11.478387, -31.571203) -> (11.485626, -31.554649)
  line L1490 (11.485626, -31.554649) -> (11.425809, -31.255964)
  line L1491 (11.425809, -31.255964) -> (11.406949, -31.213616)
  line L1492 (11.406949, -31.213616) -> (10.280332, -28.664897)
  line L1493 (10.280332, -28.664897) -> (10.260901, -28.620491)
  line L1494 (10.260901, -28.620491) -> (10.078974, -28.376556)
  line L1495 (10.078974, -28.376556) -> (10.062401, -28.371394)
  line L1496 (10.062401, -28.371394) -> (10.044875, -28.366212)
  line L1497 (10.044875, -28.366212) -> (9.740075, -28.436526)
  line L1498 (9.740075, -28.436526) -> (9.69645, -28.456147)
  line L1499 (9.69645, -28.456147) -> (9.447467, -28.566713)
  line L1500 (9.447467, -28.566713) -> (9.1861, -27.975554)
  line L1501 (9.1861, -27.975554) -> (11.655171, -26.883112)
  line L1502 (11.655171, -26.883112) -> (11.916537, -27.474272)
  line L1503 (11.916537, -27.474272) -> (11.788521, -27.531136)
  line L1504 (11.788521, -27.531136) -> (11.742991, -27.550777)
  line L1505 (11.742991, -27.550777) -> (11.482387, -27.732666)
  line L1506 (11.482387, -27.732666) -> (11.475339, -27.749202)
  line L1507 (11.475339, -27.749202) -> (11.466957, -27.765737)
  line L1508 (11.466957, -27.765737) -> (11.52506, -28.062365)
  line L1509 (11.52506, -28.062365) -> (11.54449, -28.105779)
  line L1510 (11.54449, -28.105779) -> (11.934063, -28.986347)
  line L1511 (11.934063, -28.986347) -> (13.391388, -28.340399)
  line L1512 (13.391388, -28.340399) -> (13.001815, -27.460861)
  line L1513 (13.001815, -27.460861) -> (12.982004, -27.417446)
  line L1514 (12.982004, -27.417446) -> (12.80141, -27.175587)
  line L1515 (12.80141, -27.175587) -> (12.783693, -27.170424)
  line L1516 (12.783693, -27.170424) -> (12.766167, -27.164233)
  line L1517 (12.766167, -27.164233) -> (12.456033, -27.234509)
  line L1518 (12.456033, -27.234509) -> (12.411646, -27.255178)
  line L1519 (12.411646, -27.255178) -> (12.284583, -27.311013)
  line L1520 (12.284583, -27.311013) -> (12.022836, -26.719816)
  line L1521 (12.022836, -26.719816) -> (14.492097, -25.627374)
  line L1522 (14.492097, -25.627374) -> (14.753653, -26.218534)
  line L1523 (14.753653, -26.218534) -> (14.504479, -26.329138)
  line L1524 (14.504479, -26.329138) -> (14.460093, -26.34876)
  line L1525 (14.460093, -26.34876) -> (14.199679, -26.530668)
  line L1526 (14.199679, -26.530668) -> (14.19244, -26.548232)
  line L1527 (14.19244, -26.548232) -> (14.184059, -26.564768)
  line L1528 (14.184059, -26.564768) -> (14.239875, -26.861395)
  line L1529 (14.239875, -26.861395) -> (14.259687, -26.90481)
  line L1530 (14.259687, -26.90481) -> (15.387066, -29.452462)
  line L1531 (15.387066, -29.452462) -> (15.405926, -29.494848)
  line L1532 (15.405926, -29.494848) -> (15.588805, -29.73564)
  line L1533 (15.588805, -29.73564) -> (15.606141, -29.74187)
  line L1534 (15.606141, -29.74187) -> (15.623857, -29.747032)
  line L1535 (15.623857, -29.747032) -> (15.932849, -29.677785)
  line L1536 (15.932849, -29.677785) -> (15.977426, -29.659174)
  line L1537 (15.977426, -29.659174) -> (16.226409, -29.548588)
  line L1538 (16.226409, -29.548588) -> (16.487775, -30.138738)
  line L1539 (16.487775, -30.138738) -> (14.018704, -31.23118)
  line L1540 (14.018704, -31.23118) -> (13.757339, -30.64103)
  line L1541 (13.757339, -30.64103) -> (13.885355, -30.584165)
  line L1542 (13.885355, -30.584165) -> (13.929741, -30.564544)
  line L1543 (13.929741, -30.564544) -> (14.189392, -30.382635)
  line L1544 (14.189392, -30.382635) -> (14.197584, -30.3661)
  line L1545 (14.197584, -30.3661) -> (14.205014, -30.348536)
  line L1546 (14.205014, -30.348536) -> (14.148054, -30.05088)
  line L1547 (14.148054, -30.05088) -> (14.129194, -30.008513)
  line L1548 (14.129194, -30.008513) -> (13.662279, -28.952247)
  line L1549 (13.662279, -28.952247) -> (12.204002, -29.596137)
  line L1550 (12.204002, -29.596137) -> (12.67225, -30.65446)
  line L1551 (12.67225, -30.65446) -> (12.690729, -30.696827)
  line L1552 (12.690729, -30.696827) -> (12.871514, -30.937657)
  line L1553 (12.871514, -30.937657) -> (12.88923, -30.943848)
  line L1554 (12.88923, -30.943848) -> (12.905613, -30.94903)
  line L1555 (12.905613, -30.94903) -> (13.215747, -30.879764)
  line L1556 (13.215747, -30.879764) -> (13.261276, -30.860124)
  line L1557 (13.261276, -30.860124) -> (13.389293, -30.803298)
  line L1558 (13.389293, -30.803298) -> (13.651992, -31.394457)
  line L1559 (13.651992, -31.394457) -> (11.182922, -32.486917)
  line L1560 (32.170688, -0.001143) -> (32.170688, 1.012888)
  line L1561 (32.170688, 1.012888) -> (31.915418, 4.051554)
  line L1562 (31.915418, 4.051554) -> (31.335726, 7.317295)
  line L1563 (31.335726, 7.317295) -> (31.17323, 7.953184)
  line L1564 (31.17323, 7.953184) -> (30.470475, 7.686484)
  line L1565 (30.470475, 7.686484) -> (30.625542, 7.07155)
  line L1566 (30.625542, 7.07155) -> (31.180659, 3.914013)
  line L1567 (31.180659, 3.914013) -> (31.425451, 0.977646)
  line L1568 (31.425451, 0.977646) -> (31.425451, -0.001143)
  line L1569 (31.425451, -0.001143) -> (31.425451, -0.940499)
  line L1570 (31.425451, -0.940499) -> (31.201233, -3.759899)
  line L1571 (31.201233, -3.759899) -> (30.546865, -7.388733)
  line L1572 (30.546865, -7.388733) -> (29.488638, -10.861358)
  line L1573 (29.488638, -10.861358) -> (28.051887, -14.151102)
  line L1574 (28.051887, -14.151102) -> (26.261949, -17.234154)
  line L1575 (26.261949, -17.234154) -> (24.145304, -20.08352)
  line L1576 (24.145304, -20.08352) -> (21.727859, -22.674586)
  line L1577 (21.727859, -22.674586) -> (19.738467, -24.443988)
  line L1578 (19.738467, -24.443988) -> (19.035522, -24.981427)
  line L1579 (19.035522, -24.981427) -> (19.482054, -25.578797)
  line L1580 (19.482054, -25.578797) -> (20.201382, -25.028976)
  line L1581 (20.201382, -25.028976) -> (22.238399, -23.217188)
  line L1582 (22.238399, -23.217188) -> (24.714708, -20.565161)
  line L1583 (24.714708, -20.565161) -> (26.882217, -17.647539)
  line L1584 (26.882217, -17.647539) -> (28.715589, -14.491144)
  line L1585 (28.715589, -14.491144) -> (30.187392, -11.121771)
  line L1586 (30.187392, -11.121771) -> (31.271337, -7.565517)
  line L1587 (31.271337, -7.565517) -> (31.941326, -3.850005)
  line L1588 (31.941326, -3.850005) -> (32.170688, -0.963359)
  line L1589 (32.170688, -0.963359) -> (32.170688, -0.001143)
  line L1590 (-31.425471, -0.001143) -> (-31.425471, 0.977646)
  line L1591 (-31.425471, 0.977646) -> (-31.181573, 3.914013)
  line L1592 (-31.181573, 3.914013) -> (-30.626552, 7.07155)
  line L1593 (-30.626552, 7.07155) -> (-30.470494, 7.686484)
  line L1594 (-30.470494, 7.686484) -> (-31.173287, 7.953184)
  line L1595 (-31.173287, 7.953184) -> (-31.336583, 7.317295)
  line L1596 (-31.336583, 7.317295) -> (-31.916389, 4.051554)
  line L1597 (-31.916389, 4.051554) -> (-32.17063, 1.012888)